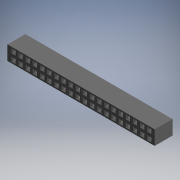
# Autodesk Inventor part: IDSD-20_lb
Saved by Autodesk Inventor 2017.3 (Build 213256000, 256)
## iProperties
Part Number: IDSD-20_lb
Material: Generic
Catalog Web Link: www.cadenas.de
Description: IDSS, IDSD Series - Lower Body-.100" Slim Body, IDC Ribbon Cable Assembly, Socket
Vendor: SAMTEC
Document SubType Name: Modeling
Designer: partserver
Manufacturer: SAMTEC
Mass: 1.32405 g
Surface Area: 26.842 cm^2
Volume: 1.32405 cm^3
Density: 1 g/cm^3
Appearance: PSOLRGB-127-127-127
Category: PARTsolutions
Company: SAMTEC
Title: IDSD-20_lb
Author: Cadenas PARTsolutions
Comments: .100" Slim Body, IDC Ribbon Cable Assembly, Socket
PSOL_IDENT_0: {$CADENAS_DATA\23d-libs\samtec\modelling\idsd\parts\idsd_lower_body.prj},194 {VTYP=3D},{NB=IDSD-20_l
PSOL_IDENT_1: b},{LINA=IDSD-20_lb},{NN=IDSS, IDSD Series - Lower Body},{DATE=12.08.2019 09:04:52},{GEOMDATE=14.12.
PSOL_IDENT_2: 2015 08:49:00},{VERSION=},{LINEID=20},{WBVAR=POS,POLOPT},{WBNUMERIC=}  {NB=IDSD-20_lb},{LINA=IDSD-20
PSOL_IDENT_3: _lb},{KT=DUMMY},{PN=IDSD-20},{SERIES=IDSD},{POS=20},{POSNO=20},{POLOPT=Not Selected},{POLOPTALG='01'
PSOL_IDENT_4: ,'02','03','04','05','06','07','08','09','10','11','12','13','14','15','16','17','18','19','20','21'
PSOL_IDENT_5: ,'22','23','24','25','26','27','28','29','30','31','32','33','34','35','36','37','38','39','40'},{PO
PSOL_IDENT_6: LOPTMAX='01','02','03','04','05','06','07','08','09','10','11','12','13','14','15','16','17','18','1
PSOL_IDENT_7: 9','20','21','22','23','24','25','26','27','28','29','30','31','32','33','34','35','36','37','38','3
PSOL_IDENT_8: 9','40','41','42','43','44','45','46','47','48','49','50','51','52','53','54','55','56','57','58','5
PSOL_IDENT_9: 9','60','61','62','63','64','65','66','67','68','69','70','71','72'},{POLOPTCTF=40},{POLOPTPN=},{POL
PSOL_IDENT_10: OPTNO=0},{ROWNO=2},{POLPLANEPOS=0},{POLPINPOS=0},{A=2.05900000},{B=0.20},{C=0.10},{D=0.365}
NB: IDSD-20_lb
NN: IDSS, IDSD Series - Lower Body
NT: .100" Slim Body, IDC Ribbon Cable Assembly, Socket
NBSYN: $PN._lb
LINA: IDSD-20_lb
CATALOG: Samtec
SERIES: IDSD
POS: -20
POLOPT: Not Selected
POLOPTMAX: '01','02','03','04','05','06','07','08','09','10','11','12','13','14','15','16','17','18','19','20','21','22','23','24','25','26','27','28','29','30','31','32','33','34','35','36','37','38','39','40','41','42','43','44','45','46','47','48','49','50','51','52','53','54','55','56','57','58','59','60','61','62','63','64','65','66','67','68','69','70','71','72'
B: 0.2
C: 0.1
SUPPLIER: SAMTEC
ARTICLENO: IDSD-20_lb
BOMINFO: IDSD-20_lb
CREATOR: CADENAS GmbH
Autodesk Inventor part; units mm, degrees
sketch "Sketch_1" plane through (0, 0, 0) normal (0, 1, 0) x (-1, 0, 0)
  line L0 (26.1493, 2.54) -> (-26.1493, 2.54)
  line L1 (-26.1493, 2.54) -> (-26.1493, -2.54)
  line L2 (-26.1493, -2.54) -> (26.1493, -2.54)
  line L3 (26.1493, -2.54) -> (26.1493, 2.54)
  line L4 (-23.6347, -0.508) -> (-25.6476, -0.508)
  line L5 (-25.6476, -0.508) -> (-25.6476, -0.889)
  line L6 (-25.6476, -0.889) -> (-24.5999, -0.889)
  line L7 (-24.5999, -0.889) -> (-24.5999, -1.651)
  line L8 (-24.5999, -1.651) -> (-23.6347, -1.651)
  line L9 (-23.6347, -1.651) -> (-23.6347, -0.508)
  line L10 (-22.3837, 0.508) -> (-22.3837, 0.889)
  line L11 (-22.3837, 0.889) -> (-23.4315, 0.889)
  line L12 (-23.4315, 0.889) -> (-23.4315, 1.651)
  line L13 (-23.4315, 1.651) -> (-24.3967, 1.651)
  line L14 (-24.3967, 1.651) -> (-24.3967, 0.508)
  line L15 (-24.3967, 0.508) -> (-22.3837, 0.508)
  line L16 (-21.0947, -0.508) -> (-23.1076, -0.508)
  line L17 (-23.1076, -0.508) -> (-23.1076, -0.889)
  line L18 (-23.1076, -0.889) -> (-22.0599, -0.889)
  line L19 (-22.0599, -0.889) -> (-22.0599, -1.651)
  line L20 (-22.0599, -1.651) -> (-21.0947, -1.651)
  line L21 (-21.0947, -1.651) -> (-21.0947, -0.508)
  line L22 (-19.8438, 0.508) -> (-19.8438, 0.889)
  line L23 (-19.8438, 0.889) -> (-20.8915, 0.889)
  line L24 (-20.8915, 0.889) -> (-20.8915, 1.651)
  line L25 (-20.8915, 1.651) -> (-21.8567, 1.651)
  line L26 (-21.8567, 1.651) -> (-21.8567, 0.508)
  line L27 (-21.8567, 0.508) -> (-19.8438, 0.508)
  line L28 (-18.5547, -0.508) -> (-20.5677, -0.508)
  line L29 (-20.5677, -0.508) -> (-20.5677, -0.889)
  line L30 (-20.5677, -0.889) -> (-19.5199, -0.889)
  line L31 (-19.5199, -0.889) -> (-19.5199, -1.651)
  line L32 (-19.5199, -1.651) -> (-18.5547, -1.651)
  line L33 (-18.5547, -1.651) -> (-18.5547, -0.508)
  line L34 (-17.3038, 0.508) -> (-17.3038, 0.889)
  line L35 (-17.3038, 0.889) -> (-18.3515, 0.889)
  line L36 (-18.3515, 0.889) -> (-18.3515, 1.651)
  line L37 (-18.3515, 1.651) -> (-19.3167, 1.651)
  line L38 (-19.3167, 1.651) -> (-19.3167, 0.508)
  line L39 (-19.3167, 0.508) -> (-17.3038, 0.508)
  line L40 (-16.0147, -0.508) -> (-18.0277, -0.508)
  line L41 (-18.0277, -0.508) -> (-18.0277, -0.889)
  line L42 (-18.0277, -0.889) -> (-16.9799, -0.889)
  line L43 (-16.9799, -0.889) -> (-16.9799, -1.651)
  line L44 (-16.9799, -1.651) -> (-16.0147, -1.651)
  line L45 (-16.0147, -1.651) -> (-16.0147, -0.508)
  line L46 (-14.7638, 0.508) -> (-14.7638, 0.889)
  line L47 (-14.7638, 0.889) -> (-15.8115, 0.889)
  line L48 (-15.8115, 0.889) -> (-15.8115, 1.651)
  line L49 (-15.8115, 1.651) -> (-16.7767, 1.651)
  line L50 (-16.7767, 1.651) -> (-16.7767, 0.508)
  line L51 (-16.7767, 0.508) -> (-14.7638, 0.508)
  line L52 (-13.4747, -0.508) -> (-15.4876, -0.508)
  line L53 (-15.4876, -0.508) -> (-15.4876, -0.889)
  line L54 (-15.4876, -0.889) -> (-14.4399, -0.889)
  line L55 (-14.4399, -0.889) -> (-14.4399, -1.651)
  line L56 (-14.4399, -1.651) -> (-13.4747, -1.651)
  line L57 (-13.4747, -1.651) -> (-13.4747, -0.508)
  line L58 (-12.2237, 0.508) -> (-12.2237, 0.889)
  line L59 (-12.2237, 0.889) -> (-13.2715, 0.889)
  line L60 (-13.2715, 0.889) -> (-13.2715, 1.651)
  line L61 (-13.2715, 1.651) -> (-14.2367, 1.651)
  line L62 (-14.2367, 1.651) -> (-14.2367, 0.508)
  line L63 (-14.2367, 0.508) -> (-12.2237, 0.508)
  line L64 (-10.9347, -0.508) -> (-12.9477, -0.508)
  line L65 (-12.9477, -0.508) -> (-12.9477, -0.889)
  line L66 (-12.9477, -0.889) -> (-11.8999, -0.889)
  line L67 (-11.8999, -0.889) -> (-11.8999, -1.651)
  line L68 (-11.8999, -1.651) -> (-10.9347, -1.651)
  line L69 (-10.9347, -1.651) -> (-10.9347, -0.508)
  line L70 (-9.6837, 0.508) -> (-9.6837, 0.889)
  line L71 (-9.6837, 0.889) -> (-10.7315, 0.889)
  line L72 (-10.7315, 0.889) -> (-10.7315, 1.651)
  line L73 (-10.7315, 1.651) -> (-11.6967, 1.651)
  line L74 (-11.6967, 1.651) -> (-11.6967, 0.508)
  line L75 (-11.6967, 0.508) -> (-9.6837, 0.508)
  line L76 (-8.3947, -0.508) -> (-10.4077, -0.508)
  line L77 (-10.4077, -0.508) -> (-10.4077, -0.889)
  line L78 (-10.4077, -0.889) -> (-9.3599, -0.889)
  line L79 (-9.3599, -0.889) -> (-9.3599, -1.651)
  line L80 (-9.3599, -1.651) -> (-8.3947, -1.651)
  line L81 (-8.3947, -1.651) -> (-8.3947, -0.508)
  line L82 (-7.1437, 0.508) -> (-7.1437, 0.889)
  line L83 (-7.1437, 0.889) -> (-8.1915, 0.889)
  line L84 (-8.1915, 0.889) -> (-8.1915, 1.651)
  line L85 (-8.1915, 1.651) -> (-9.1567, 1.651)
  line L86 (-9.1567, 1.651) -> (-9.1567, 0.508)
  line L87 (-9.1567, 0.508) -> (-7.1437, 0.508)
  line L88 (-5.8547, -0.508) -> (-7.8677, -0.508)
  line L89 (-7.8677, -0.508) -> (-7.8677, -0.889)
  line L90 (-7.8677, -0.889) -> (-6.8199, -0.889)
  line L91 (-6.8199, -0.889) -> (-6.8199, -1.651)
  line L92 (-6.8199, -1.651) -> (-5.8547, -1.651)
  line L93 (-5.8547, -1.651) -> (-5.8547, -0.508)
  line L94 (-4.6037, 0.508) -> (-4.6037, 0.889)
  line L95 (-4.6037, 0.889) -> (-5.6515, 0.889)
  line L96 (-5.6515, 0.889) -> (-5.6515, 1.651)
  line L97 (-5.6515, 1.651) -> (-6.6167, 1.651)
  line L98 (-6.6167, 1.651) -> (-6.6167, 0.508)
  line L99 (-6.6167, 0.508) -> (-4.6037, 0.508)
  line L100 (-3.3147, -0.508) -> (-5.3276, -0.508)
  line L101 (-5.3276, -0.508) -> (-5.3276, -0.889)
  line L102 (-5.3276, -0.889) -> (-4.2799, -0.889)
  line L103 (-4.2799, -0.889) -> (-4.2799, -1.651)
  line L104 (-4.2799, -1.651) -> (-3.3147, -1.651)
  line L105 (-3.3147, -1.651) -> (-3.3147, -0.508)
  line L106 (-2.0638, 0.508) -> (-2.0638, 0.889)
  line L107 (-2.0638, 0.889) -> (-3.1115, 0.889)
  line L108 (-3.1115, 0.889) -> (-3.1115, 1.651)
  line L109 (-3.1115, 1.651) -> (-4.0767, 1.651)
  line L110 (-4.0767, 1.651) -> (-4.0767, 0.508)
  line L111 (-4.0767, 0.508) -> (-2.0638, 0.508)
  line L112 (-0.7747, -0.508) -> (-2.7876, -0.508)
  line L113 (-2.7876, -0.508) -> (-2.7876, -0.889)
  line L114 (-2.7876, -0.889) -> (-1.7399, -0.889)
  line L115 (-1.7399, -0.889) -> (-1.7399, -1.651)
  line L116 (-1.7399, -1.651) -> (-0.7747, -1.651)
  line L117 (-0.7747, -1.651) -> (-0.7747, -0.508)
  line L118 (0.4763, 0.508) -> (0.4763, 0.889)
  line L119 (0.4763, 0.889) -> (-0.5715, 0.889)
  line L120 (-0.5715, 0.889) -> (-0.5715, 1.651)
  line L121 (-0.5715, 1.651) -> (-1.5367, 1.651)
  line L122 (-1.5367, 1.651) -> (-1.5367, 0.508)
  line L123 (-1.5367, 0.508) -> (0.4763, 0.508)
  line L124 (1.7653, -0.508) -> (-0.2476, -0.508)
  line L125 (-0.2476, -0.508) -> (-0.2476, -0.889)
  line L126 (-0.2476, -0.889) -> (0.8001, -0.889)
  line L127 (0.8001, -0.889) -> (0.8001, -1.651)
  line L128 (0.8001, -1.651) -> (1.7653, -1.651)
  line L129 (1.7653, -1.651) -> (1.7653, -0.508)
  line L130 (3.0162, 0.508) -> (3.0162, 0.889)
  line L131 (3.0162, 0.889) -> (1.9685, 0.889)
  line L132 (1.9685, 0.889) -> (1.9685, 1.651)
  line L133 (1.9685, 1.651) -> (1.0033, 1.651)
  line L134 (1.0033, 1.651) -> (1.0033, 0.508)
  line L135 (1.0033, 0.508) -> (3.0162, 0.508)
  line L136 (4.3053, -0.508) -> (2.2923, -0.508)
  line L137 (2.2923, -0.508) -> (2.2923, -0.889)
  line L138 (2.2923, -0.889) -> (3.3401, -0.889)
  line L139 (3.3401, -0.889) -> (3.3401, -1.651)
  line L140 (3.3401, -1.651) -> (4.3053, -1.651)
  line L141 (4.3053, -1.651) -> (4.3053, -0.508)
  line L142 (5.5563, 0.508) -> (5.5563, 0.889)
  line L143 (5.5563, 0.889) -> (4.5085, 0.889)
  line L144 (4.5085, 0.889) -> (4.5085, 1.651)
  line L145 (4.5085, 1.651) -> (3.5433, 1.651)
  line L146 (3.5433, 1.651) -> (3.5433, 0.508)
  line L147 (3.5433, 0.508) -> (5.5563, 0.508)
  line L148 (6.8453, -0.508) -> (4.8323, -0.508)
  line L149 (4.8323, -0.508) -> (4.8323, -0.889)
  line L150 (4.8323, -0.889) -> (5.8801, -0.889)
  line L151 (5.8801, -0.889) -> (5.8801, -1.651)
  line L152 (5.8801, -1.651) -> (6.8453, -1.651)
  line L153 (6.8453, -1.651) -> (6.8453, -0.508)
  line L154 (8.0962, 0.508) -> (8.0962, 0.889)
  line L155 (8.0962, 0.889) -> (7.0485, 0.889)
  line L156 (7.0485, 0.889) -> (7.0485, 1.651)
  line L157 (7.0485, 1.651) -> (6.0833, 1.651)
  line L158 (6.0833, 1.651) -> (6.0833, 0.508)
  line L159 (6.0833, 0.508) -> (8.0962, 0.508)
  line L160 (9.3853, -0.508) -> (7.3724, -0.508)
  line L161 (7.3724, -0.508) -> (7.3724, -0.889)
  line L162 (7.3724, -0.889) -> (8.4201, -0.889)
  line L163 (8.4201, -0.889) -> (8.4201, -1.651)
  line L164 (8.4201, -1.651) -> (9.3853, -1.651)
  line L165 (9.3853, -1.651) -> (9.3853, -0.508)
  line L166 (10.6363, 0.508) -> (10.6363, 0.889)
  line L167 (10.6363, 0.889) -> (9.5885, 0.889)
  line L168 (9.5885, 0.889) -> (9.5885, 1.651)
  line L169 (9.5885, 1.651) -> (8.6233, 1.651)
  line L170 (8.6233, 1.651) -> (8.6233, 0.508)
  line L171 (8.6233, 0.508) -> (10.6363, 0.508)
  line L172 (11.9253, -0.508) -> (9.9123, -0.508)
  line L173 (9.9123, -0.508) -> (9.9123, -0.889)
  line L174 (9.9123, -0.889) -> (10.9601, -0.889)
  line L175 (10.9601, -0.889) -> (10.9601, -1.651)
  line L176 (10.9601, -1.651) -> (11.9253, -1.651)
  line L177 (11.9253, -1.651) -> (11.9253, -0.508)
  line L178 (13.1762, 0.508) -> (13.1762, 0.889)
  line L179 (13.1762, 0.889) -> (12.1285, 0.889)
  line L180 (12.1285, 0.889) -> (12.1285, 1.651)
  line L181 (12.1285, 1.651) -> (11.1633, 1.651)
  line L182 (11.1633, 1.651) -> (11.1633, 0.508)
  line L183 (11.1633, 0.508) -> (13.1762, 0.508)
  line L184 (14.4653, -0.508) -> (12.4524, -0.508)
  line L185 (12.4524, -0.508) -> (12.4524, -0.889)
  line L186 (12.4524, -0.889) -> (13.5001, -0.889)
  line L187 (13.5001, -0.889) -> (13.5001, -1.651)
  line L188 (13.5001, -1.651) -> (14.4653, -1.651)
  line L189 (14.4653, -1.651) -> (14.4653, -0.508)
  line L190 (15.7163, 0.508) -> (15.7163, 0.889)
  line L191 (15.7163, 0.889) -> (14.6685, 0.889)
  line L192 (14.6685, 0.889) -> (14.6685, 1.651)
  line L193 (14.6685, 1.651) -> (13.7033, 1.651)
  line L194 (13.7033, 1.651) -> (13.7033, 0.508)
  line L195 (13.7033, 0.508) -> (15.7163, 0.508)
  line L196 (17.0053, -0.508) -> (14.9924, -0.508)
  line L197 (14.9924, -0.508) -> (14.9924, -0.889)
  line L198 (14.9924, -0.889) -> (16.0401, -0.889)
  line L199 (16.0401, -0.889) -> (16.0401, -1.651)
  line L200 (16.0401, -1.651) -> (17.0053, -1.651)
  line L201 (17.0053, -1.651) -> (17.0053, -0.508)
  line L202 (18.2563, 0.508) -> (18.2563, 0.889)
  line L203 (18.2563, 0.889) -> (17.2085, 0.889)
  line L204 (17.2085, 0.889) -> (17.2085, 1.651)
  line L205 (17.2085, 1.651) -> (16.2433, 1.651)
  line L206 (16.2433, 1.651) -> (16.2433, 0.508)
  line L207 (16.2433, 0.508) -> (18.2563, 0.508)
  line L208 (19.5453, -0.508) -> (17.5324, -0.508)
  line L209 (17.5324, -0.508) -> (17.5324, -0.889)
  line L210 (17.5324, -0.889) -> (18.5801, -0.889)
  line L211 (18.5801, -0.889) -> (18.5801, -1.651)
  line L212 (18.5801, -1.651) -> (19.5453, -1.651)
  line L213 (19.5453, -1.651) -> (19.5453, -0.508)
  line L214 (20.7963, 0.508) -> (20.7963, 0.889)
  line L215 (20.7963, 0.889) -> (19.7485, 0.889)
  line L216 (19.7485, 0.889) -> (19.7485, 1.651)
  line L217 (19.7485, 1.651) -> (18.7833, 1.651)
  line L218 (18.7833, 1.651) -> (18.7833, 0.508)
  line L219 (18.7833, 0.508) -> (20.7963, 0.508)
  line L220 (22.0853, -0.508) -> (20.0724, -0.508)
  line L221 (20.0724, -0.508) -> (20.0724, -0.889)
  line L222 (20.0724, -0.889) -> (21.1201, -0.889)
  line L223 (21.1201, -0.889) -> (21.1201, -1.651)
  line L224 (21.1201, -1.651) -> (22.0853, -1.651)
  line L225 (22.0853, -1.651) -> (22.0853, -0.508)
  line L226 (23.3362, 0.508) -> (23.3362, 0.889)
  line L227 (23.3362, 0.889) -> (22.2885, 0.889)
  line L228 (22.2885, 0.889) -> (22.2885, 1.651)
  line L229 (22.2885, 1.651) -> (21.3233, 1.651)
  line L230 (21.3233, 1.651) -> (21.3233, 0.508)
  line L231 (21.3233, 0.508) -> (23.3362, 0.508)
  line L232 (24.6253, -0.508) -> (22.6123, -0.508)
  line L233 (22.6123, -0.508) -> (22.6123, -0.889)
  line L234 (22.6123, -0.889) -> (23.6601, -0.889)
  line L235 (23.6601, -0.889) -> (23.6601, -1.651)
  line L236 (23.6601, -1.651) -> (24.6253, -1.651)
  line L237 (24.6253, -1.651) -> (24.6253, -0.508)
  line L238 (25.8762, 0.508) -> (25.8762, 0.889)
  line L239 (25.8762, 0.889) -> (24.8285, 0.889)
  line L240 (24.8285, 0.889) -> (24.8285, 1.651)
  line L241 (24.8285, 1.651) -> (23.8633, 1.651)
  line L242 (23.8633, 1.651) -> (23.8633, 0.508)
  line L243 (23.8633, 0.508) -> (25.8762, 0.508)
  constraints: 488 end point
extrude "Extrusion1" add sketch "Sketch_1" along normal blind 6.35
sketch "Sketch_3" plane through (0, 0, 0) normal (0, 1, 0) x (-1, 0, 0)
  line L0 (26.1493, 2.54) -> (-26.1493, 2.54)
  line L1 (-26.1493, 2.54) -> (-26.1493, -2.54)
  line L2 (-26.1493, -2.54) -> (26.1493, -2.54)
  line L3 (26.1493, -2.54) -> (26.1493, 2.54)
  line L4 (-23.6347, -1.651) -> (-23.6347, -0.889)
  line L5 (-23.6347, -0.889) -> (-24.3967, -0.889)
  line L6 (-24.3967, -0.889) -> (-24.3967, -1.651)
  line L7 (-24.3967, -1.651) -> (-23.6347, -1.651)
  line L8 (-23.6347, 0.889) -> (-23.6347, 1.651)
  line L9 (-23.6347, 1.651) -> (-24.3967, 1.651)
  line L10 (-24.3967, 1.651) -> (-24.3967, 0.889)
  line L11 (-24.3967, 0.889) -> (-23.6347, 0.889)
  line L12 (-21.0947, -1.651) -> (-21.0947, -0.889)
  line L13 (-21.0947, -0.889) -> (-21.8567, -0.889)
  line L14 (-21.8567, -0.889) -> (-21.8567, -1.651)
  line L15 (-21.8567, -1.651) -> (-21.0947, -1.651)
  line L16 (-21.0947, 0.889) -> (-21.0947, 1.651)
  line L17 (-21.0947, 1.651) -> (-21.8567, 1.651)
  line L18 (-21.8567, 1.651) -> (-21.8567, 0.889)
  line L19 (-21.8567, 0.889) -> (-21.0947, 0.889)
  line L20 (-18.5547, -1.651) -> (-18.5547, -0.889)
  line L21 (-18.5547, -0.889) -> (-19.3167, -0.889)
  line L22 (-19.3167, -0.889) -> (-19.3167, -1.651)
  line L23 (-19.3167, -1.651) -> (-18.5547, -1.651)
  line L24 (-18.5547, 0.889) -> (-18.5547, 1.651)
  line L25 (-18.5547, 1.651) -> (-19.3167, 1.651)
  line L26 (-19.3167, 1.651) -> (-19.3167, 0.889)
  line L27 (-19.3167, 0.889) -> (-18.5547, 0.889)
  line L28 (-16.0147, -1.651) -> (-16.0147, -0.889)
  line L29 (-16.0147, -0.889) -> (-16.7767, -0.889)
  line L30 (-16.7767, -0.889) -> (-16.7767, -1.651)
  line L31 (-16.7767, -1.651) -> (-16.0147, -1.651)
  line L32 (-16.0147, 0.889) -> (-16.0147, 1.651)
  line L33 (-16.0147, 1.651) -> (-16.7767, 1.651)
  line L34 (-16.7767, 1.651) -> (-16.7767, 0.889)
  line L35 (-16.7767, 0.889) -> (-16.0147, 0.889)
  line L36 (-13.4747, -1.651) -> (-13.4747, -0.889)
  line L37 (-13.4747, -0.889) -> (-14.2367, -0.889)
  line L38 (-14.2367, -0.889) -> (-14.2367, -1.651)
  line L39 (-14.2367, -1.651) -> (-13.4747, -1.651)
  line L40 (-13.4747, 0.889) -> (-13.4747, 1.651)
  line L41 (-13.4747, 1.651) -> (-14.2367, 1.651)
  line L42 (-14.2367, 1.651) -> (-14.2367, 0.889)
  line L43 (-14.2367, 0.889) -> (-13.4747, 0.889)
  line L44 (-10.9347, -1.651) -> (-10.9347, -0.889)
  line L45 (-10.9347, -0.889) -> (-11.6967, -0.889)
  line L46 (-11.6967, -0.889) -> (-11.6967, -1.651)
  line L47 (-11.6967, -1.651) -> (-10.9347, -1.651)
  line L48 (-10.9347, 0.889) -> (-10.9347, 1.651)
  line L49 (-10.9347, 1.651) -> (-11.6967, 1.651)
  line L50 (-11.6967, 1.651) -> (-11.6967, 0.889)
  line L51 (-11.6967, 0.889) -> (-10.9347, 0.889)
  line L52 (-8.3947, -1.651) -> (-8.3947, -0.889)
  line L53 (-8.3947, -0.889) -> (-9.1567, -0.889)
  line L54 (-9.1567, -0.889) -> (-9.1567, -1.651)
  line L55 (-9.1567, -1.651) -> (-8.3947, -1.651)
  line L56 (-8.3947, 0.889) -> (-8.3947, 1.651)
  line L57 (-8.3947, 1.651) -> (-9.1567, 1.651)
  line L58 (-9.1567, 1.651) -> (-9.1567, 0.889)
  line L59 (-9.1567, 0.889) -> (-8.3947, 0.889)
  line L60 (-5.8547, -1.651) -> (-5.8547, -0.889)
  line L61 (-5.8547, -0.889) -> (-6.6167, -0.889)
  line L62 (-6.6167, -0.889) -> (-6.6167, -1.651)
  line L63 (-6.6167, -1.651) -> (-5.8547, -1.651)
  line L64 (-5.8547, 0.889) -> (-5.8547, 1.651)
  line L65 (-5.8547, 1.651) -> (-6.6167, 1.651)
  line L66 (-6.6167, 1.651) -> (-6.6167, 0.889)
  line L67 (-6.6167, 0.889) -> (-5.8547, 0.889)
  line L68 (-3.3147, -1.651) -> (-3.3147, -0.889)
  line L69 (-3.3147, -0.889) -> (-4.0767, -0.889)
  line L70 (-4.0767, -0.889) -> (-4.0767, -1.651)
  line L71 (-4.0767, -1.651) -> (-3.3147, -1.651)
  line L72 (-3.3147, 0.889) -> (-3.3147, 1.651)
  line L73 (-3.3147, 1.651) -> (-4.0767, 1.651)
  line L74 (-4.0767, 1.651) -> (-4.0767, 0.889)
  line L75 (-4.0767, 0.889) -> (-3.3147, 0.889)
  line L76 (-0.7747, -1.651) -> (-0.7747, -0.889)
  line L77 (-0.7747, -0.889) -> (-1.5367, -0.889)
  line L78 (-1.5367, -0.889) -> (-1.5367, -1.651)
  line L79 (-1.5367, -1.651) -> (-0.7747, -1.651)
  line L80 (-0.7747, 0.889) -> (-0.7747, 1.651)
  line L81 (-0.7747, 1.651) -> (-1.5367, 1.651)
  line L82 (-1.5367, 1.651) -> (-1.5367, 0.889)
  line L83 (-1.5367, 0.889) -> (-0.7747, 0.889)
  line L84 (1.7653, -1.651) -> (1.7653, -0.889)
  line L85 (1.7653, -0.889) -> (1.0033, -0.889)
  line L86 (1.0033, -0.889) -> (1.0033, -1.651)
  line L87 (1.0033, -1.651) -> (1.7653, -1.651)
  line L88 (1.7653, 0.889) -> (1.7653, 1.651)
  line L89 (1.7653, 1.651) -> (1.0033, 1.651)
  line L90 (1.0033, 1.651) -> (1.0033, 0.889)
  line L91 (1.0033, 0.889) -> (1.7653, 0.889)
  line L92 (4.3053, -1.651) -> (4.3053, -0.889)
  line L93 (4.3053, -0.889) -> (3.5433, -0.889)
  line L94 (3.5433, -0.889) -> (3.5433, -1.651)
  line L95 (3.5433, -1.651) -> (4.3053, -1.651)
  line L96 (4.3053, 0.889) -> (4.3053, 1.651)
  line L97 (4.3053, 1.651) -> (3.5433, 1.651)
  line L98 (3.5433, 1.651) -> (3.5433, 0.889)
  line L99 (3.5433, 0.889) -> (4.3053, 0.889)
  line L100 (6.8453, -1.651) -> (6.8453, -0.889)
  line L101 (6.8453, -0.889) -> (6.0833, -0.889)
  line L102 (6.0833, -0.889) -> (6.0833, -1.651)
  line L103 (6.0833, -1.651) -> (6.8453, -1.651)
  line L104 (6.8453, 0.889) -> (6.8453, 1.651)
  line L105 (6.8453, 1.651) -> (6.0833, 1.651)
  line L106 (6.0833, 1.651) -> (6.0833, 0.889)
  line L107 (6.0833, 0.889) -> (6.8453, 0.889)
  line L108 (9.3853, -1.651) -> (9.3853, -0.889)
  line L109 (9.3853, -0.889) -> (8.6233, -0.889)
  line L110 (8.6233, -0.889) -> (8.6233, -1.651)
  line L111 (8.6233, -1.651) -> (9.3853, -1.651)
  line L112 (9.3853, 0.889) -> (9.3853, 1.651)
  line L113 (9.3853, 1.651) -> (8.6233, 1.651)
  line L114 (8.6233, 1.651) -> (8.6233, 0.889)
  line L115 (8.6233, 0.889) -> (9.3853, 0.889)
  line L116 (11.9253, -1.651) -> (11.9253, -0.889)
  line L117 (11.9253, -0.889) -> (11.1633, -0.889)
  line L118 (11.1633, -0.889) -> (11.1633, -1.651)
  line L119 (11.1633, -1.651) -> (11.9253, -1.651)
  line L120 (11.9253, 0.889) -> (11.9253, 1.651)
  line L121 (11.9253, 1.651) -> (11.1633, 1.651)
  line L122 (11.1633, 1.651) -> (11.1633, 0.889)
  line L123 (11.1633, 0.889) -> (11.9253, 0.889)
  line L124 (14.4653, -1.651) -> (14.4653, -0.889)
  line L125 (14.4653, -0.889) -> (13.7033, -0.889)
  line L126 (13.7033, -0.889) -> (13.7033, -1.651)
  line L127 (13.7033, -1.651) -> (14.4653, -1.651)
  line L128 (14.4653, 0.889) -> (14.4653, 1.651)
  line L129 (14.4653, 1.651) -> (13.7033, 1.651)
  line L130 (13.7033, 1.651) -> (13.7033, 0.889)
  line L131 (13.7033, 0.889) -> (14.4653, 0.889)
  line L132 (17.0053, -1.651) -> (17.0053, -0.889)
  line L133 (17.0053, -0.889) -> (16.2433, -0.889)
  line L134 (16.2433, -0.889) -> (16.2433, -1.651)
  line L135 (16.2433, -1.651) -> (17.0053, -1.651)
  line L136 (17.0053, 0.889) -> (17.0053, 1.651)
  line L137 (17.0053, 1.651) -> (16.2433, 1.651)
  line L138 (16.2433, 1.651) -> (16.2433, 0.889)
  line L139 (16.2433, 0.889) -> (17.0053, 0.889)
  line L140 (19.5453, -1.651) -> (19.5453, -0.889)
  line L141 (19.5453, -0.889) -> (18.7833, -0.889)
  line L142 (18.7833, -0.889) -> (18.7833, -1.651)
  line L143 (18.7833, -1.651) -> (19.5453, -1.651)
  line L144 (19.5453, 0.889) -> (19.5453, 1.651)
  line L145 (19.5453, 1.651) -> (18.7833, 1.651)
  line L146 (18.7833, 1.651) -> (18.7833, 0.889)
  line L147 (18.7833, 0.889) -> (19.5453, 0.889)
  line L148 (22.0853, -1.651) -> (22.0853, -0.889)
  line L149 (22.0853, -0.889) -> (21.3233, -0.889)
  line L150 (21.3233, -0.889) -> (21.3233, -1.651)
  line L151 (21.3233, -1.651) -> (22.0853, -1.651)
  line L152 (22.0853, 0.889) -> (22.0853, 1.651)
  line L153 (22.0853, 1.651) -> (21.3233, 1.651)
  line L154 (21.3233, 1.651) -> (21.3233, 0.889)
  line L155 (21.3233, 0.889) -> (22.0853, 0.889)
  line L156 (24.6253, -1.651) -> (24.6253, -0.889)
  line L157 (24.6253, -0.889) -> (23.8633, -0.889)
  line L158 (23.8633, -0.889) -> (23.8633, -1.651)
  line L159 (23.8633, -1.651) -> (24.6253, -1.651)
  line L160 (24.6253, 0.889) -> (24.6253, 1.651)
  line L161 (24.6253, 1.651) -> (23.8633, 1.651)
  line L162 (23.8633, 1.651) -> (23.8633, 0.889)
  line L163 (23.8633, 0.889) -> (24.6253, 0.889)
  constraints: 328 end point
extrude "Extrusion2" add sketch "Sketch_3" along normal blind 0.889
sketch "Sketch_4" plane through (0, 0, 0) normal (0, 1, 0) x (-1, 0, 0)
  line L0 (25.0063, 0.508) -> (25.0063, 2.032)
  line L1 (25.0063, 2.032) -> (23.4823, 2.032)
  line L2 (23.4823, 2.032) -> (23.4823, 0.508)
  line L3 (23.4823, 0.508) -> (25.0063, 0.508)
  constraints: 8 end point
extrude "Extrusion3" cut sketch "Sketch_4" along normal blind 0.4572 draft -39.8
pattern_linear "Rectangular Pattern1" count 20 spacing 2.54 along (1, 0, 0) of "Extrusion3"
sketch "Sketch_7" plane through (0, 0, 0) normal (0, 1, 0) x (-1, 0, 0)
  line L0 (25.0063, -0.508) -> (23.4823, -0.508)
  line L1 (23.4823, -0.508) -> (23.4823, -2.032)
  line L2 (23.4823, -2.032) -> (25.0063, -2.032)
  line L3 (25.0063, -2.032) -> (25.0063, -0.508)
  constraints: 8 end point
extrude "Extrusion4" cut sketch "Sketch_7" along normal blind 0.4572 draft -39.8
pattern_linear "Rectangular Pattern2" count 20 spacing 2.54 along (1, 0, 0) of "Extrusion4"
ref_plane "lower_body_to_cable_XY" through (0, 6.7945, 0) normal (0, 1, 0) x (1, 0, 0)
ref_plane "lower_body_to_cable_YZ" through (0, 6.7945, 0) normal (1, 0, 0) x (0, 0, -1)
ref_plane "lower_body_to_cable_ZX" through (0, 6.7945, 0) normal (0, 0, -1) x (0, 1, 0)
ref_plane "lower_body_to_dummy_XY" through (0, 0, 0) normal (0, 1, 0) x (1, 0, 0)
ref_plane "lower_body_to_dummy_YZ" through (0, 0, 0) normal (1, 0, 0) x (0, 0, -1)
ref_plane "lower_body_to_dummy_ZX" through (0, 0, 0) normal (0, 0, -1) x (0, 1, 0)
ref_plane "lower_body_to_dummy_reverse_XY" through (0, 0, 0) normal (0, -1, 0) x (1, 0, 0)
ref_plane "lower_body_to_dummy_reverse_YZ" through (0, 0, 0) normal (1, 0, 0) x (0, 0, 1)
ref_plane "lower_body_to_dummy_reverse_ZX" through (0, 0, 0) normal (0, 0, 1) x (0, -1, 0)
ref_plane "lower_body_to_upper_body_XY" through (0, 9.271, 0) normal (0, 1, 0) x (1, 0, 0)
ref_plane "lower_body_to_upper_body_YZ" through (0, 9.271, 0) normal (1, 0, 0) x (0, 0, -1)
ref_plane "lower_body_to_upper_body_ZX" through (0, 9.271, 0) normal (0, 0, -1) x (0, 1, 0)
ref_plane "lower_body_to_upper_body_reverse_XY" through (0, 9.271, 0) normal (0, -1, 0) x (1, 0, 0)
ref_plane "lower_body_to_upper_body_reverse_YZ" through (0, 9.271, 0) normal (1, 0, 0) x (0, 0, 1)
ref_plane "lower_body_to_upper_body_reverse_ZX" through (0, 9.271, 0) normal (0, 0, 1) x (0, -1, 0)
ref_plane "pin_XY" through (-24.2443, 1.016, 1.27) normal (0, 1, 0) x (1, 0, 0)
ref_plane "pin_YZ" through (-24.2443, 1.016, 1.27) normal (1, 0, 0) x (0, 0, -1)
ref_plane "pin_ZX" through (-24.2443, 1.016, 1.27) normal (0, 0, -1) x (0, 1, 0)
ref_plane "pin2_XY" through (24.0157, 1.016, -1.27) normal (0, 1, 0) x (1, 0, 0)
ref_plane "pin2_YZ" through (24.0157, 1.016, -1.27) normal (1, 0, 0) x (0, 0, -1)
ref_plane "pin2_ZX" through (24.0157, 1.016, -1.27) normal (0, 0, -1) x (0, 1, 0)
ref_plane "pin2_reverse_XY" through (24.0157, 1.016, -1.27) normal (0, -1, 0) x (1, 0, 0)
ref_plane "pin2_reverse_YZ" through (24.0157, 1.016, -1.27) normal (1, 0, 0) x (0, 0, 1)
ref_plane "pin2_reverse_ZX" through (24.0157, 1.016, -1.27) normal (0, 0, 1) x (0, -1, 0)
ref_plane "pin_reverse_XY" through (-24.2443, 1.016, 1.27) normal (0, -1, 0) x (1, 0, 0)
ref_plane "pin_reverse_YZ" through (-24.2443, 1.016, 1.27) normal (1, 0, 0) x (0, 0, 1)
ref_plane "pin_reverse_ZX" through (-24.2443, 1.016, 1.27) normal (0, 0, 1) x (0, -1, 0)
body "Solid1"
